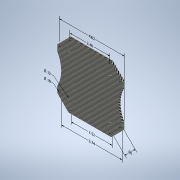
# Autodesk Inventor part: F450_GPS_mount.
Saved by Autodesk Inventor 2020.1 (Build 241239000, 239)
## iProperties
Created: 2019-12-02
Part Number: F450_GPS_mount.
Material: CFRP
Document SubType Name: Modeling
Designer: makhi
Density: 1.43 g/cm^3
Appearance: Carbon Fiber
Author: makhi
Autodesk Inventor part; units mm, degrees
ref_plane "YZ Plane" through (0, 0, 0) normal (1, 0, 0) x (0, 1, 0)
ref_plane "XZ Plane" through (0, 0, 0) normal (0, 1, 0) x (-1, 0, 0)
ref_plane "XY Plane" through (0, 0, 0) normal (0, 0, 1) x (1, 0, 0)
sketch "Sketch3" plane through (0, 0, 0) normal (0, 0, 1) x (1, 0, 0)
  line L0 (50.9998, -51.0001) -> (-50.9998, -51.0001)
  line L1 (-50.9998, -51.0001) -> (-50.9998, 51.0001)
  line L2 (-50.9998, 51.0001) -> (50.9998, 51.0001)
  line L3 (50.9998, 51.0001) -> (50.9998, -51.0001)
  line L4 (50.9998, -51.0001) -> (-50.9998, 51.0001) construction
  line L5 (-50.9998, -51.0001) -> (50.9998, 51.0001) construction
  point P0 (0, 0)
  dimension "d2" = 101.9996
  dimension "d3" = 102.0002
  constraints: 12 end point, 2 midpoint, 2 parallel, 1 horizontal, 1 perpendicular
  measures "d2" distance of L1.end L2.end
  measures "d3" distance of L2.end L0.start
sketch "Sketch7" plane through (0, 0, 0) normal (0, 0, 1) x (1, 0, 0)
  circle A0 centre (32.0004, 32.0005) radius 1.5002
  circle A1 centre (-31.9991, 32.0005) radius 1.5002
  circle A2 centre (-31.999, 32.0005) radius 1.5002
  circle A3 centre (-31.9991, -32.0002) radius 1.5002
  circle A4 centre (-31.999, -32.0002) radius 1.5002
  circle A5 centre (32.0003, -32.0002) radius 1.5002
  circle A6 centre (32.0004, -32.0002) radius 1.5002
  constraints: 7 centre point
extrude "Extrusion2" add sketch "Sketch3" along normal blind 3
hole "Hole1" at (-31.999, -32.0002, 0) at (-31.999, 32.0005, 0) at (32.0004, 32.0005, 0) at (32.0004, -32.0002, 0) direction (0, 0, 1) diameter 3 end through all countersink diameter 3.0226 countersink angle 82
sketch "Sketch8" plane through (0, 0, 0) normal (0, 0, -1) x (-1, 0, 0)
  circle A0 centre (47.5, 31.25) radius 1.2502
  circle A1 centre (31.25, 47.5) radius 1.2502
  circle A2 centre (-47.5, -31.25) radius 1.2502
  circle A3 centre (-31.25, -47.5) radius 1.2502
  circle A4 centre (-47.5, 31.25) radius 1.2502
  circle A5 centre (-31.25, 47.5) radius 1.2502
  circle A6 centre (47.5, -31.25) radius 1.2502
  circle A7 centre (31.25, -47.5) radius 1.2502
  constraints: 8 centre point
hole "Hole2" at (47.5, -31.25, 0) at (31.25, -47.5, 0) at (-31.25, -47.5, 0) at (-47.5, -31.25, 0) at (47.5, 31.25, 0) at (31.25, 47.5, 0) at (-31.25, 47.5, 0) at (-47.5, 31.25, 0) direction (0, 0, 1) diameter 2.5 end through all countersink diameter 2.6 countersink angle 82
sketch "Sketch9" plane through (0, 0, 0) normal (0, 0, -1) x (-1, 0, 0)
  point P0 (0, 0)
sketch "Sketch10" plane through (0, 0, 0) normal (0, 0, -1) x (-1, 0, 0)
  point P0 (0, 0)
sketch "Sketch11" plane through (0, 0, 0) normal (0, 0, -1) x (-1, 0, 0)
  line L0 (68.6779, 50.7734) -> (50.9999, 33.0954)
  line L1 (50.9999, 33.0954) -> (33.3221, 50.7732)
  line L2 (33.3221, 50.7732) -> (51.0001, 68.4512)
  line L3 (51.0001, 68.4512) -> (68.6779, 50.7734)
  line L4 (68.6779, 50.7734) -> (33.3221, 50.7732) construction
  line L5 (50.9999, 33.0954) -> (51.0001, 68.4512) construction
  line L6 (-33.3221, 50.7734) -> (-51.0001, 33.0954)
  line L7 (-51.0001, 33.0954) -> (-68.6779, 50.7732)
  line L8 (-68.6779, 50.7732) -> (-50.9999, 68.4512)
  line L9 (-50.9999, 68.4512) -> (-33.3221, 50.7734)
  line L10 (-33.3221, 50.7734) -> (-68.6779, 50.7732) construction
  line L11 (-51.0001, 33.0954) -> (-50.9999, 68.4512) construction
  line L12 (-33.3221, -51.2266) -> (-51.0001, -68.9046)
  line L13 (-51.0001, -68.9046) -> (-68.6779, -51.2268)
  line L14 (-68.6779, -51.2268) -> (-50.9999, -33.5488)
  line L15 (-50.9999, -33.5488) -> (-33.3221, -51.2266)
  line L16 (-33.3221, -51.2266) -> (-68.6779, -51.2268) construction
  line L17 (-51.0001, -68.9046) -> (-50.9999, -33.5488) construction
  line L18 (68.6779, -51.2266) -> (50.9999, -68.9046)
  line L19 (50.9999, -68.9046) -> (33.3221, -51.2268)
  line L20 (33.3221, -51.2268) -> (51.0001, -33.5488)
  line L21 (51.0001, -33.5488) -> (68.6779, -51.2266)
  line L22 (68.6779, -51.2266) -> (33.3221, -51.2268) construction
  line L23 (50.9999, -68.9046) -> (51.0001, -33.5488) construction
  point P0 (51, 50.7733)
  point P1 (-51, 50.7733)
  point P2 (-51, -51.2267)
  point P3 (51, -51.2267)
  constraints: 48 end point, 8 midpoint, 8 parallel, 4 perpendicular
extrude "Extrusion3" cut sketch "Sketch11" against normal blind 3
sketch "Sketch12" plane through (0, 0, 0) normal (0, 0, -1) x (-1, 0, 0)
  line L0 (-50.9998, -33.5489) -> (-50.9998, 33.0957) projected
  arc A0 (-50.9998, -22.9999) -> (-50.9998, 22.9999) centre (-92.056, 0) ccw
  line L1 (-50.9998, 22.9999) -> (-50.9998, -22.9999)
  arc A1 (51.0009, 22.9999) -> (51.0009, -22.9999) centre (92.0571, 0) ccw
  line L2 (51.0009, -22.9999) -> (51.0009, 22.9999)
  point P0 (0, 0)
  constraints: 4 end point, 4 point on circle, 2 centre point, 2 point on line, 1 collinear
extrude "Extrusion4" cut sketch "Sketch12" against normal blind 3
body "Solid2"
